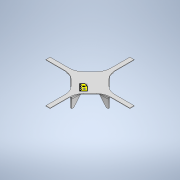
# Autodesk Inventor part: frame
Saved by Autodesk Inventor 2020 (Build 240168000, 168)
## iProperties
Created: 2020-01-05
Part Number: frame
Material: Generic
Document SubType Name: Modeling
Designer: gp190
Density: 1 g/cm^3
Appearance: Default
Author: gp190
Autodesk Inventor part; units mm, degrees
ref_plane "YZ Plane" through (0, 0, 0) normal (1, 0, 0) x (0, 1, 0)
ref_plane "XZ Plane" through (0, 0, 0) normal (0, 1, 0) x (-1, 0, 0)
ref_plane "XY Plane" through (0, 0, 0) normal (0, 0, 1) x (1, 0, 0)
sketch "base" plane through (0, 0, 0) normal (0, 1, 0) x (-1, 0, 0)
  line L0 (38.7382, 75.5618) -> (75.5618, 38.7382)
  line L1 (75.5618, -38.7382) -> (38.7382, -75.5618)
  line L2 (-38.7382, 75.5618) -> (-75.5618, 38.7382)
  line L3 (-75.5619, -38.7377) -> (-38.7387, -75.5604)
  line L4 (12.7, 138.4236) -> (12.7, 254)
  line L5 (12.7, 254) -> (-12.7, 254)
  line L6 (-12.7, 254) -> (-12.7, 138.4236)
  line L7 (-138.4236, 12.7) -> (-254, 12.7)
  line L8 (-254, 12.7) -> (-254, -12.7)
  line L9 (-254, -12.7) -> (-138.4232, -12.7)
  line L10 (-12.7, -138.4227) -> (-12.7, -254)
  line L11 (-12.7, -254) -> (12.7, -254)
  line L12 (12.7, -254) -> (12.7, -138.4236)
  line L13 (138.4236, -12.7) -> (254, -12.7)
  line L14 (254, -12.7) -> (254, 12.7)
  line L15 (254, 12.7) -> (138.4236, 12.7)
  arc A0 (12.7, 138.4236) -> (38.7382, 75.5618) centre (101.6, 138.4236) ccw
  arc A1 (75.5618, 38.7382) -> (138.4236, 12.7) centre (138.4236, 101.6) ccw
  arc A2 (138.4236, -12.7) -> (75.5618, -38.7382) centre (138.4236, -101.6) ccw
  arc A3 (38.7382, -75.5618) -> (12.7, -138.4236) centre (101.6, -138.4236) ccw
  arc A4 (-12.7, -138.4227) -> (-38.7387, -75.5604) centre (-101.6, -138.4227) ccw
  arc A5 (-138.4236, 12.7) -> (-75.5618, 38.7382) centre (-138.4236, 101.6) ccw
  arc A6 (-38.7382, 75.5618) -> (-12.7, 138.4236) centre (-101.6, 138.4236) ccw
  arc A7 (-75.5619, -38.7377) -> (-138.4232, -12.7) centre (-138.4232, -101.6) ccw
  point P0 (0, 0)
  constraints: 32 end point, 16 point on circle, 16 tangent, 8 centre point, 8 perpendicular, 5 equal radius, 2 horizontal, 2 vertical
extrude "Extrusion1" add sketch "base" along normal mid plane 2.54
sketch "Sketch10" plane through (0, 0, 0) normal (1, 0, 0) x (0, 1, 0)
  line L0 (0, 38.1) -> (-76.2, 101.6)
  line L1 (-76.2, 101.6) -> (-76.2, 114.3)
  line L2 (-76.2, 114.3) -> (0, 114.3)
  line L3 (0, 114.3) -> (0, 38.1)
  line L4 (-76.2, -101.6) -> (-76.2, -114.3)
  line L5 (0, -114.3) -> (0, -38.1)
  line L6 (0, -38.1) -> (-76.2, -101.6)
  line L7 (0, -114.3) -> (-76.2, -114.3)
  point P0 (0, 0)
  constraints: 16 end point, 1 horizontal, 1 perpendicular
sketch "Sketch12" plane through (0, 0, 0) normal (0, 0, 1) x (1, 0, 0)
  line L0 (-38.1, 0) -> (-101.6, -76.2)
  line L1 (-101.6, -76.2) -> (-114.3, -76.2)
  line L2 (-114.3, -76.2) -> (-114.3, 0)
  line L3 (-114.3, 0) -> (-38.1, 0)
  line L4 (101.6, -76.2) -> (114.3, -76.2)
  line L5 (114.3, 0) -> (38.1, 0)
  line L6 (38.1, 0) -> (101.6, -76.2)
  line L7 (114.3, 0) -> (114.3, -76.2)
  point P0 (0, 0)
  point P1 (0, 0)
  constraints: 16 end point, 1 perpendicular
extrude "Estrusion4" add sketch "Sketch10" along normal mid plane 7.62 contours L0 L1 L2 L3
extrude "Extrusion5" add sketch "Sketch10" against normal mid plane 7.62 contours L6 L5 L7 L4
extrude "Extrusion6" add sketch "Sketch12" along normal mid plane 7.62 contours L0 L1 L2 L3
extrude "Extrusion7" add sketch "Sketch12" along normal mid plane 7.62 contours L6 L5 L7 L4
fillet "Fillet4" radius 25.4 12 edges at (-3.81, -1.27, 76.7292) (3.81, -1.27, 76.7292) (-76.7292, -1.27, 3.81) (0, -1.27, 39.1583) (-39.1583, -1.27, 0) (-76.7292, -1.27, -3.81) (-3.81, -1.27, -76.7292) (0, -1.27, -39.1583) (39.1583, -1.27, 0) (76.7292, -1.27, -3.81) (76.7292, -1.27, 3.81) (3.81, -1.27, -76.7292)
fillet "Fillet5" radius 25.4 4 edges at (-0.0001, -1.27, -114.3) (-114.3, -1.27, 0) (0, -1.27, 114.3) (114.3, -1.27, 0.0001)
body "Solid1"
